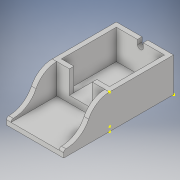
# Autodesk Inventor part: Holster
Saved by Autodesk Inventor 2018 (Build 220112000, 112)
## iProperties
Created: 2018-01-15
Part Number: Holster
Material: Generic
Document SubType Name: Modeling
Designer: Mandus
Density: 1 g/cm^3
Appearance: Default
Author: Mandus
Autodesk Inventor part; units mm, degrees
ref_plane "YZ Plane" through (0, 0, 0) normal (1, 0, 0) x (0, 1, 0)
ref_plane "XZ Plane" through (0, 0, 0) normal (0, 1, 0) x (-1, 0, 0)
ref_plane "XY Plane" through (0, 0, 0) normal (0, 0, 1) x (1, 0, 0)
sketch "Sketch1" plane through (0, 0, 0) normal (0, 1, 0) x (-1, 0, 0)
  line L0 (0, 0) -> (25, 0)
  line L1 (25, 0) -> (25, -28)
  line L2 (25, -28) -> (0, -28)
  line L3 (0, -28) -> (0, 0)
  dimension "d0" = 25
  dimension "d1" = 28
  constraints: 8 end point, 2 parallel, 1 horizontal, 1 perpendicular
  measures "d0" distance of L1.end L2.end
  measures "d1" distance of L0.end L1.end
extrude "Extrusion1" add sketch "Sketch1" along normal blind 15
sketch "Sketch2" plane through (0, 15, 0) normal (0, 1, 0) x (1, 0, 0)
  point P0 (0, 0)
shell "Shell1" thickness 2 removed faces 1 at (-8.3333, 15, -9.3333)
sketch "Sketch3" plane through (0, 0, 0) normal (1, 0, 0) x (0, 0, -1)
  point P0 (0, 0)
sketch "Sketch4" plane through (0, 0, 0) normal (1, 0, 0) x (0, 0, -1)
  line L0 (0, 0) -> (0, 15) projected
  line L1 (0, 15) -> (0, 0)
  line L2 (0, 0) -> (-20, 0)
  line L3 (-20, 0) -> (-20, 2)
  arc A0 (-19, 3) -> (-20, 2) centre (-19, 2) ccw
  arc A1 (-19, 3) -> (-9.089, 9.2596) centre (-19, 13.976) ccw
  line L4 (28, 15) -> (0, 15) projected
  arc A2 (0, 15) -> (-9.089, 9.2596) centre (0, 4.9343) ccw
  line L5 (0, 15) -> (28, 15) projected
  dimension "d5" = 20
  dimension "d6" = 2
  dimension "d7" = 1
  constraints: 6 end point, 6 point on circle, 4 tangent, 3 centre point, 1 horizontal, 1 perpendicular, 1 vertical
  measures "d5" distance of L0.start L2.end
  measures "d6" distance of L2.end L3.end
  measures "d7" radius of A0
extrude "Extrusion2" add sketch "Sketch4" against normal blind 25
sketch "Sketch5" plane through (0, 0, -28) normal (0, 0, -1) x (-1, 0, 0)
  circle A0 centre (12.5, 13) radius 1.25
  line L0 (11.25, 13) -> (11.25, 15)
  line L1 (0, 15) -> (25, 15) projected
  line L2 (11.25, 15) -> (13.75, 15)
  line L3 (13.75, 15) -> (13.75, 13)
  point P0 (0, 0)
  dimension "d10" = 2.5
  constraints: 6 end point, 2 point on circle, 1 centre point, 1 horizontal, 1 perpendicular, 1 point on line, 1 vertical
  measures "d10" diameter of A0
sketch "Sketch6" plane through (0, 0, -28) normal (0, 0, -1) x (-1, 0, 0)
  point P0 (0, 0)
extrude "Extrusion3" cut sketch "Sketch5" against normal up to next
sketch "Sketch7" plane through (-23, 2, -2) normal (0, 1, 0) x (1, 0, 0)
  point P0 (23, -2)
sketch "Sketch8" plane through (0, 15, 0) normal (0, 1, 0) x (1, 0, 0)
  line L0 (-2, 0) -> (-23, 0)
  line L1 (-23, 0) -> (-23, -20)
  line L2 (-23, -20) -> (-2, -20)
  line L3 (-2, -20) -> (-2, 0)
  line L4 (-12.5, 0) -> (-7.5, 0)
  line L5 (-7.5, 0) -> (-7.5, 2)
  line L6 (-7.5, 2) -> (-12.5, 2)
  line L7 (-12.5, 2) -> (-12.5, 0)
  line L8 (-12.5, 0) -> (-17.5, 0)
  line L9 (-17.5, 0) -> (-17.5, 2)
  line L10 (-17.5, 2) -> (-12.5, 2)
  line L11 (-12.5, 2) -> (-12.5, 0)
  point P0 (0, 0)
  dimension "d13" = 21
  dimension "d14" = 20
  dimension "d15" = 5
  dimension "d16" = 2
  dimension "d17" = 5
  dimension "d18" = 2
  constraints: 24 end point, 6 parallel, 3 horizontal, 3 perpendicular, 1 midpoint
  measures "d13" distance of L2.end L1.end
  measures "d14" distance of L1.end L0.end
  measures "d15" distance of L6.end L5.end
  measures "d16" distance of L5.end L4.end
  measures "d17" distance of L9.end L10.end
  measures "d18" distance of L8.end L9.end
extrude "Extrusion4" cut sketch "Sketch8" against normal up to surface (13 mm away) contours L3 L2 L1 L0
extrude "Extrusion5" cut sketch "Sketch8" against normal blind 10 contours L0 L7 L6 L5 | L0 L9 L10 L7
sketch "Sketch9" plane through (-23, 2, -2) normal (0, 1, 0) x (1, 0, 0)
  line L0 (5.5, 0) -> (15.5, 0) projected
  line L1 (5.5, 0) -> (15.5, 0)
  line L2 (15.5, 0) -> (15.5, 10)
  line L3 (15.5, 10) -> (5.5, 10)
  line L4 (5.5, 10) -> (5.5, 0)
  point P0 (23, -2)
  dimension "d23" = 10
  dimension "d24" = 10
  constraints: 8 end point, 2 parallel, 1 horizontal, 1 perpendicular
  measures "d23" distance of L3.end L2.end
  measures "d24" distance of L2.end L1.end
extrude "Extrusion6" add sketch "Sketch9" along normal up to surface (3 mm away)
body "Solid1"
